Autodesk Fusion 360 part; units mm, degrees
(part 2 of 2)
  constraint coincident L91.end L95
  constraint collinear L91 L92
  constraint collinear L93 L94
  constraint coincident L95.end L99
  constraint collinear L95 L96
  constraint collinear L97 L98
  constraint collinear L99 L100
  constraint coincident L102.start L107
  constraint collinear L101 L102
  constraint coincident L104.start L105
  constraint collinear L103 L104
  constraint collinear L105 L106
  constraint collinear L107 L108
  constraint collinear L109 L110
  constraint collinear L111 L112
  constraint collinear L113 L114
  constraint perpendicular L35 L115
  constraint perpendicular L36 L116
  constraint collinear L341 L342
  constraint coincident L344.start L349
  constraint collinear L343 L344
  constraint coincident L346.start L347
  constraint collinear L345 L346
  constraint collinear L347 L348
  constraint collinear L349 L350
  constraint coincident L351.end L355
  constraint collinear L351 L352
  constraint collinear L353 L354
  constraint coincident L355.end L367
  constraint collinear L355 L356
  constraint coincident L358.start L365
  constraint collinear L357 L358
  constraint coincident L360.start L361
  constraint collinear L359 L360
  constraint coincident A101.end L361
  constraint collinear L361 L362
  constraint collinear L363 L364
  constraint collinear L365 L366
  constraint collinear L367 L368
  constraint coincident L370.start L375
  constraint collinear L369 L370
  constraint coincident L372.start L373
  constraint collinear L371 L372
  constraint collinear L373 L374
  constraint collinear L375 L376
  constraint collinear L377 L378
  constraint coincident L379.end L383
  constraint collinear L379 L380
  constraint coincident L381.end L385
  constraint collinear L381 L382
  constraint collinear L383 L384
  constraint collinear L385 L386
  constraint collinear L387 L388
  constraint coincident L388.start L395
  constraint collinear L389 L390
  constraint coincident L392.start L393
  constraint collinear L391 L392
  constraint collinear L393 L394
  constraint collinear L395 L396
  constraint coincident L398.start L403
  constraint collinear L397 L398
  constraint coincident L400.start L401
  constraint collinear L399 L400
  constraint collinear L401 L402
  constraint collinear L403 L404
  constraint coincident L405.end L409
  constraint collinear L405 L406
  constraint collinear L407 L408
  constraint coincident L409.end L413
  constraint collinear L409 L410
  constraint collinear L411 L412
  constraint collinear L413 L414
  constraint coincident L416.start L423
  constraint collinear L415 L416
  constraint coincident L418.start L421
  constraint collinear L417 L418
  constraint collinear L419 L420
  constraint collinear L421 L422
  constraint collinear L423 L424
  measures "d74" distance of L342.end L352.end
  measures "d82" distance of L341 L355
  measures "d88" diameter of A100
  measures "d89" diameter of A99
  measures "d93" distance of L349 L367
  measures "d95" distance of L341.start L342.end
  measures "d98" distance of A100.centre L367
  measures "d103" distance of L341 L343
  measures "d104" diameter of A97
  measures "d105" diameter of A98
  measures "d106" diameter of A96
  measures "d107" distance of A96.centre L341
  measures "d113" distance of L3.start L3.end
sketch "Schizzo17" plane through (0, 0, 16) normal (0, 0, 1) x (-1, 0, 0) in component "Cubo"
  line L0 (-47.5456, -19.25) -> (-48.649, -19.25)
  arc A0 (-48.649, -18.05) -> (-48.649, -19.25) centre (-49.7456, -18.65) ccw
  line L1 (-48.649, -18.05) -> (-47.5456, -18.05)
  line L2 (-47.5456, -18.05) -> (-47.5456, -12.5)
  line L3 (-47.5456, -12.5) -> (-46.2956, -12.5)
  line L4 (-46.2956, -12.5) -> (-46.2956, -10.9)
  line L5 (-46.2956, -10.9) -> (-48.649, -10.9)
  arc A1 (-48.649, -9.7) -> (-48.649, -10.9) centre (-49.7456, -10.3) ccw
  line L6 (-48.649, -9.7) -> (-46.2956, -9.7)
  line L7 (-46.2956, -9.7) -> (-46.2956, -8.9715)
  arc A2 (-43.6956, -8.9715) -> (-46.2956, -8.9715) centre (-44.9956, -7.8) ccw
  line L8 (-43.6956, -8.9715) -> (-43.6956, -9.7)
  line L9 (-43.6956, -9.7) -> (-41.3421, -9.7)
  arc A3 (-41.3421, -10.9) -> (-41.3421, -9.7) centre (-40.2456, -10.3) ccw
  line L10 (-41.3421, -10.9) -> (-43.6956, -10.9)
  line L11 (-43.6956, -10.9) -> (-43.6956, -12.5)
  line L12 (-43.6956, -12.5) -> (-42.4456, -12.5)
  line L13 (-42.4456, -12.5) -> (-42.4456, -18.05)
  line L14 (-42.4456, -18.05) -> (-41.3421, -18.05)
  arc A4 (-41.3421, -19.25) -> (-41.3421, -18.05) centre (-40.2456, -18.65) ccw
  line L15 (-41.3421, -19.25) -> (-42.4456, -19.25)
  line L16 (-42.4456, -19.25) -> (-42.4456, -24.8)
  line L17 (-42.4456, -24.8) -> (-43.6956, -24.8)
  line L18 (-43.6956, -24.8) -> (-43.6956, -26.4)
  line L19 (-43.6956, -26.4) -> (-41.3421, -26.4)
  arc A5 (-41.3421, -27.6) -> (-41.3421, -26.4) centre (-40.2456, -27) ccw
  line L20 (-41.3421, -27.6) -> (-43.6956, -27.6)
  line L21 (-43.6956, -27.6) -> (-43.6956, -28.3285)
  arc A6 (-46.2956, -28.3285) -> (-43.6956, -28.3285) centre (-44.9956, -29.5) ccw
  line L22 (-46.2956, -28.3285) -> (-46.2956, -27.6)
  line L23 (-46.2956, -27.6) -> (-48.649, -27.6)
  arc A7 (-48.649, -26.4) -> (-48.649, -27.6) centre (-49.7456, -27) ccw
  line L24 (-48.649, -26.4) -> (-46.2956, -26.4)
  line L25 (-46.2956, -26.4) -> (-46.2956, -24.8)
  line L26 (-46.2956, -24.8) -> (-47.5456, -24.8)
  line L27 (-47.5456, -24.8) -> (-47.5456, -19.25)
  arc A8 (-27.7171, -37.25) -> (-27.7171, -36.05) centre (-26.6206, -36.65) ccw
  line L28 (-27.7171, -37.25) -> (-30.0706, -37.25)
  line L29 (-30.0706, -37.25) -> (-30.0706, -38.85)
  line L30 (-30.0706, -38.85) -> (-28.8206, -38.85)
  line L31 (-28.8206, -38.85) -> (-28.8206, -44.4)
  line L32 (-28.8206, -44.4) -> (-27.7171, -44.4)
  arc A9 (-27.7171, -45.6) -> (-27.7171, -44.4) centre (-26.6206, -45) ccw
  line L33 (-27.7171, -45.6) -> (-28.8206, -45.6)
  line L34 (-28.8206, -45.6) -> (-28.8206, -51.15)
  line L35 (-28.8206, -51.15) -> (-30.0706, -51.15)
  line L36 (-30.0706, -51.15) -> (-30.0706, -52.75)
  line L37 (-30.0706, -52.75) -> (-27.7171, -52.75)
  arc A10 (-27.7171, -53.95) -> (-27.7171, -52.75) centre (-26.6206, -53.35) ccw
  line L38 (-27.7171, -53.95) -> (-30.0706, -53.95)
  line L39 (-30.0706, -53.95) -> (-30.0706, -54.6785)
  arc A11 (-32.6706, -54.6785) -> (-30.0706, -54.6785) centre (-31.3706, -55.85) ccw
  line L40 (-32.6706, -54.6785) -> (-32.6706, -53.95)
  line L41 (-32.6706, -53.95) -> (-35.024, -53.95)
  arc A12 (-35.024, -52.75) -> (-35.024, -53.95) centre (-36.1206, -53.35) ccw
  line L42 (-35.024, -52.75) -> (-32.6706, -52.75)
  line L43 (-32.6706, -52.75) -> (-32.6706, -51.15)
  line L44 (-32.6706, -51.15) -> (-33.9206, -51.15)
  line L45 (-33.9206, -51.15) -> (-33.9206, -45.6)
  line L46 (-33.9206, -45.6) -> (-35.024, -45.6)
  arc A13 (-35.024, -44.4) -> (-35.024, -45.6) centre (-36.1206, -45) ccw
  line L47 (-35.024, -44.4) -> (-33.9206, -44.4)
  line L48 (-33.9206, -44.4) -> (-33.9206, -38.85)
  line L49 (-33.9206, -38.85) -> (-32.6706, -38.85)
  line L50 (-32.6706, -38.85) -> (-32.6706, -37.25)
  line L51 (-32.6706, -37.25) -> (-35.024, -37.25)
  arc A14 (-35.024, -36.05) -> (-35.024, -37.25) centre (-36.1206, -36.65) ccw
  line L52 (-35.024, -36.05) -> (-32.6706, -36.05)
  line L53 (-32.6706, -36.05) -> (-32.6706, -35.3215)
  arc A15 (-30.0706, -35.3215) -> (-32.6706, -35.3215) centre (-31.3706, -34.15) ccw
  line L54 (-30.0706, -35.3215) -> (-30.0706, -36.05)
  line L55 (-30.0706, -36.05) -> (-27.7171, -36.05)
  line L56 (-70.9456, -79.1) -> (-68.5921, -79.1)
  arc A16 (-68.5921, -80.3) -> (-68.5921, -79.1) centre (-67.4956, -79.7) ccw
  line L57 (-68.5921, -80.3) -> (-70.9456, -80.3)
  line L58 (-70.9456, -80.3) -> (-70.9456, -81.0285)
  arc A17 (-73.5456, -81.0285) -> (-70.9456, -81.0285) centre (-72.2456, -82.2) ccw
  line L59 (-73.5456, -81.0285) -> (-73.5456, -80.3)
  line L60 (-73.5456, -80.3) -> (-75.899, -80.3)
  arc A18 (-75.899, -79.1) -> (-75.899, -80.3) centre (-76.9956, -79.7) ccw
  line L61 (-75.899, -79.1) -> (-73.5456, -79.1)
  line L62 (-73.5456, -79.1) -> (-73.5456, -77.5)
  line L63 (-73.5456, -77.5) -> (-74.7956, -77.5)
  line L64 (-74.7956, -77.5) -> (-74.7956, -71.95)
  line L65 (-74.7956, -71.95) -> (-75.899, -71.95)
  arc A19 (-75.899, -70.75) -> (-75.899, -71.95) centre (-76.9956, -71.35) ccw
  line L66 (-75.899, -70.75) -> (-74.7956, -70.75)
  line L67 (-74.7956, -70.75) -> (-74.7956, -65.2)
  line L68 (-74.7956, -65.2) -> (-73.5456, -65.2)
  line L69 (-73.5456, -65.2) -> (-73.5456, -63.6)
  line L70 (-73.5456, -63.6) -> (-75.899, -63.6)
  arc A20 (-75.899, -62.4) -> (-75.899, -63.6) centre (-76.9956, -63) ccw
  line L71 (-75.899, -62.4) -> (-73.5456, -62.4)
  line L72 (-73.5456, -62.4) -> (-73.5456, -61.6715)
  arc A21 (-70.9456, -61.6715) -> (-73.5456, -61.6715) centre (-72.2456, -60.5) ccw
  line L73 (-70.9456, -61.6715) -> (-70.9456, -62.4)
  line L74 (-70.9456, -62.4) -> (-68.5921, -62.4)
  arc A22 (-68.5921, -63.6) -> (-68.5921, -62.4) centre (-67.4956, -63) ccw
  line L75 (-68.5921, -63.6) -> (-70.9456, -63.6)
  line L76 (-70.9456, -63.6) -> (-70.9456, -65.2)
  line L77 (-70.9456, -65.2) -> (-69.6956, -65.2)
  line L78 (-69.6956, -65.2) -> (-69.6956, -70.75)
  line L79 (-69.6956, -70.75) -> (-68.5921, -70.75)
  arc A23 (-68.5921, -71.95) -> (-68.5921, -70.75) centre (-67.4956, -71.35) ccw
  line L80 (-68.5921, -71.95) -> (-69.6956, -71.95)
  line L81 (-69.6956, -71.95) -> (-69.6956, -77.5)
  line L82 (-69.6956, -77.5) -> (-70.9456, -77.5)
  line L83 (-70.9456, -77.5) -> (-70.9456, -79.1)
  line L84 (-15.1956, -70.75) -> (-14.0921, -70.75)
  arc A24 (-14.0921, -71.95) -> (-14.0921, -70.75) centre (-12.9956, -71.35) ccw
  line L85 (-14.0921, -71.95) -> (-15.1956, -71.95)
  line L86 (-15.1956, -71.95) -> (-15.1956, -77.5)
  line L87 (-15.1956, -77.5) -> (-16.4456, -77.5)
  line L88 (-16.4456, -77.5) -> (-16.4456, -79.1)
  line L89 (-16.4456, -79.1) -> (-14.0921, -79.1)
  arc A25 (-14.0921, -80.3) -> (-14.0921, -79.1) centre (-12.9956, -79.7) ccw
  line L90 (-14.0921, -80.3) -> (-16.4456, -80.3)
  line L91 (-16.4456, -80.3) -> (-16.4456, -81.0285)
  arc A26 (-19.0456, -81.0285) -> (-16.4456, -81.0285) centre (-17.7456, -82.2) ccw
  line L92 (-19.0456, -81.0285) -> (-19.0456, -80.3)
  line L93 (-19.0456, -80.3) -> (-21.399, -80.3)
  arc A27 (-21.399, -79.1) -> (-21.399, -80.3) centre (-22.4956, -79.7) ccw
  line L94 (-21.399, -79.1) -> (-19.0456, -79.1)
  line L95 (-19.0456, -79.1) -> (-19.0456, -77.5)
  line L96 (-19.0456, -77.5) -> (-20.2956, -77.5)
  line L97 (-20.2956, -77.5) -> (-20.2956, -71.95)
  line L98 (-20.2956, -71.95) -> (-21.399, -71.95)
  arc A28 (-21.399, -70.75) -> (-21.399, -71.95) centre (-22.4956, -71.35) ccw
  line L99 (-21.399, -70.75) -> (-20.2956, -70.75)
  line L100 (-20.2956, -70.75) -> (-20.2956, -65.2)
  line L101 (-20.2956, -65.2) -> (-19.0456, -65.2)
  line L102 (-19.0456, -65.2) -> (-19.0456, -63.6)
  line L103 (-19.0456, -63.6) -> (-21.399, -63.6)
  arc A29 (-21.399, -62.4) -> (-21.399, -63.6) centre (-22.4956, -63) ccw
  line L104 (-21.399, -62.4) -> (-19.0456, -62.4)
  line L105 (-19.0456, -62.4) -> (-19.0456, -61.6715)
  arc A30 (-16.4456, -61.6715) -> (-19.0456, -61.6715) centre (-17.7456, -60.5) ccw
  line L106 (-16.4456, -61.6715) -> (-16.4456, -62.4)
  line L107 (-16.4456, -62.4) -> (-14.0921, -62.4)
  arc A31 (-14.0921, -63.6) -> (-14.0921, -62.4) centre (-12.9956, -63) ccw
  line L108 (-14.0921, -63.6) -> (-16.4456, -63.6)
  line L109 (-16.4456, -63.6) -> (-16.4456, -65.2)
  line L110 (-16.4456, -65.2) -> (-15.1956, -65.2)
  line L111 (-15.1956, -65.2) -> (-15.1956, -70.75)
  line L112 (-57.3206, -62.4) -> (-54.9671, -62.4)
  arc A32 (-54.9671, -63.6) -> (-54.9671, -62.4) centre (-53.8706, -63) ccw
  line L113 (-54.9671, -63.6) -> (-57.3206, -63.6)
  line L114 (-57.3206, -63.6) -> (-57.3206, -65.2)
  line L115 (-57.3206, -65.2) -> (-56.0706, -65.2)
  line L116 (-56.0706, -65.2) -> (-56.0706, -70.75)
  line L117 (-56.0706, -70.75) -> (-54.9671, -70.75)
  arc A33 (-54.9671, -71.95) -> (-54.9671, -70.75) centre (-53.8706, -71.35) ccw
  line L118 (-54.9671, -71.95) -> (-56.0706, -71.95)
  line L119 (-56.0706, -71.95) -> (-56.0706, -77.5)
  line L120 (-56.0706, -77.5) -> (-57.3206, -77.5)
  line L121 (-57.3206, -77.5) -> (-57.3206, -79.1)
  line L122 (-57.3206, -79.1) -> (-54.9671, -79.1)
  arc A34 (-54.9671, -80.3) -> (-54.9671, -79.1) centre (-53.8706, -79.7) ccw
  line L123 (-54.9671, -80.3) -> (-57.3206, -80.3)
  line L124 (-57.3206, -80.3) -> (-57.3206, -81.0285)
  arc A35 (-59.9206, -81.0285) -> (-57.3206, -81.0285) centre (-58.6206, -82.2) ccw
  line L125 (-59.9206, -81.0285) -> (-59.9206, -80.3)
  line L126 (-59.9206, -80.3) -> (-62.274, -80.3)
  arc A36 (-62.274, -79.1) -> (-62.274, -80.3) centre (-63.3706, -79.7) ccw
  line L127 (-62.274, -79.1) -> (-59.9206, -79.1)
  line L128 (-59.9206, -79.1) -> (-59.9206, -77.5)
  line L129 (-59.9206, -77.5) -> (-61.1706, -77.5)
  line L130 (-61.1706, -77.5) -> (-61.1706, -71.95)
  line L131 (-61.1706, -71.95) -> (-62.274, -71.95)
  arc A37 (-62.274, -70.75) -> (-62.274, -71.95) centre (-63.3706, -71.35) ccw
  line L132 (-62.274, -70.75) -> (-61.1706, -70.75)
  line L133 (-61.1706, -70.75) -> (-61.1706, -65.2)
  line L134 (-61.1706, -65.2) -> (-59.9206, -65.2)
  line L135 (-59.9206, -65.2) -> (-59.9206, -63.6)
  line L136 (-59.9206, -63.6) -> (-62.274, -63.6)
  arc A38 (-62.274, -62.4) -> (-62.274, -63.6) centre (-63.3706, -63) ccw
  line L137 (-62.274, -62.4) -> (-59.9206, -62.4)
  line L138 (-59.9206, -62.4) -> (-59.9206, -61.6715)
  arc A39 (-57.3206, -61.6715) -> (-59.9206, -61.6715) centre (-58.6206, -60.5) ccw
  line L139 (-57.3206, -61.6715) -> (-57.3206, -62.4)
  line L140 (-47.5456, -45.6) -> (-48.649, -45.6)
  arc A40 (-48.649, -44.4) -> (-48.649, -45.6) centre (-49.7456, -45) ccw
  line L141 (-48.649, -44.4) -> (-47.5456, -44.4)
  line L142 (-47.5456, -44.4) -> (-47.5456, -38.85)
  line L143 (-47.5456, -38.85) -> (-46.2956, -38.85)
  line L144 (-46.2956, -38.85) -> (-46.2956, -37.25)
  line L145 (-46.2956, -37.25) -> (-48.649, -37.25)
  arc A41 (-48.649, -36.05) -> (-48.649, -37.25) centre (-49.7456, -36.65) ccw
  line L146 (-48.649, -36.05) -> (-46.2956, -36.05)
  line L147 (-46.2956, -36.05) -> (-46.2956, -35.3215)
  arc A42 (-43.6956, -35.3215) -> (-46.2956, -35.3215) centre (-44.9956, -34.15) ccw
  line L148 (-43.6956, -35.3215) -> (-43.6956, -36.05)
  line L149 (-43.6956, -36.05) -> (-41.3421, -36.05)
  arc A43 (-41.3421, -37.25) -> (-41.3421, -36.05) centre (-40.2456, -36.65) ccw
  line L150 (-41.3421, -37.25) -> (-43.6956, -37.25)
  line L151 (-43.6956, -37.25) -> (-43.6956, -38.85)
  line L152 (-43.6956, -38.85) -> (-42.4456, -38.85)
  line L153 (-42.4456, -38.85) -> (-42.4456, -44.4)
  line L154 (-42.4456, -44.4) -> (-41.3421, -44.4)
  arc A44 (-41.3421, -45.6) -> (-41.3421, -44.4) centre (-40.2456, -45) ccw
  line L155 (-41.3421, -45.6) -> (-42.4456, -45.6)
  line L156 (-42.4456, -45.6) -> (-42.4456, -51.15)
  line L157 (-42.4456, -51.15) -> (-43.6956, -51.15)
  line L158 (-43.6956, -51.15) -> (-43.6956, -52.75)
  line L159 (-43.6956, -52.75) -> (-41.3421, -52.75)
  arc A45 (-41.3421, -53.95) -> (-41.3421, -52.75) centre (-40.2456, -53.35) ccw
  line L160 (-41.3421, -53.95) -> (-43.6956, -53.95)
  line L161 (-43.6956, -53.95) -> (-43.6956, -54.6785)
  arc A46 (-46.2956, -54.6785) -> (-43.6956, -54.6785) centre (-44.9956, -55.85) ccw
  line L162 (-46.2956, -54.6785) -> (-46.2956, -53.95)
  line L163 (-46.2956, -53.95) -> (-48.649, -53.95)
  arc A47 (-48.649, -52.75) -> (-48.649, -53.95) centre (-49.7456, -53.35) ccw
  line L164 (-48.649, -52.75) -> (-46.2956, -52.75)
  line L165 (-46.2956, -52.75) -> (-46.2956, -51.15)
  line L166 (-46.2956, -51.15) -> (-47.5456, -51.15)
  line L167 (-47.5456, -51.15) -> (-47.5456, -45.6)
  arc A48 (-27.7171, -10.9) -> (-27.7171, -9.7) centre (-26.6206, -10.3) ccw
  line L168 (-27.7171, -10.9) -> (-30.0706, -10.9)
  line L169 (-30.0706, -10.9) -> (-30.0706, -12.5)
  line L170 (-30.0706, -12.5) -> (-28.8206, -12.5)
  line L171 (-28.8206, -12.5) -> (-28.8206, -18.05)
  line L172 (-28.8206, -18.05) -> (-27.7171, -18.05)
  arc A49 (-27.7171, -19.25) -> (-27.7171, -18.05) centre (-26.6206, -18.65) ccw
  line L173 (-27.7171, -19.25) -> (-28.8206, -19.25)
  line L174 (-28.8206, -19.25) -> (-28.8206, -24.8)
  line L175 (-28.8206, -24.8) -> (-30.0706, -24.8)
  line L176 (-30.0706, -24.8) -> (-30.0706, -26.4)
  line L177 (-30.0706, -26.4) -> (-27.7171, -26.4)
  arc A50 (-27.7171, -27.6) -> (-27.7171, -26.4) centre (-26.6206, -27) ccw
  line L178 (-27.7171, -27.6) -> (-30.0706, -27.6)
  line L179 (-30.0706, -27.6) -> (-30.0706, -28.3285)
  arc A51 (-32.6706, -28.3285) -> (-30.0706, -28.3285) centre (-31.3706, -29.5) ccw
  line L180 (-32.6706, -28.3285) -> (-32.6706, -27.6)
  line L181 (-32.6706, -27.6) -> (-35.024, -27.6)
  arc A52 (-35.024, -26.4) -> (-35.024, -27.6) centre (-36.1206, -27) ccw
  line L182 (-35.024, -26.4) -> (-32.6706, -26.4)
  line L183 (-32.6706, -26.4) -> (-32.6706, -24.8)
  line L184 (-32.6706, -24.8) -> (-33.9206, -24.8)
  line L185 (-33.9206, -24.8) -> (-33.9206, -19.25)
  line L186 (-33.9206, -19.25) -> (-35.024, -19.25)
  arc A53 (-35.024, -18.05) -> (-35.024, -19.25) centre (-36.1206, -18.65) ccw
  line L187 (-35.024, -18.05) -> (-33.9206, -18.05)
  line L188 (-33.9206, -18.05) -> (-33.9206, -12.5)
  line L189 (-33.9206, -12.5) -> (-32.6706, -12.5)
  line L190 (-32.6706, -12.5) -> (-32.6706, -10.9)
  line L191 (-32.6706, -10.9) -> (-35.024, -10.9)
  arc A54 (-35.024, -9.7) -> (-35.024, -10.9) centre (-36.1206, -10.3) ccw
  line L192 (-35.024, -9.7) -> (-32.6706, -9.7)
  line L193 (-32.6706, -9.7) -> (-32.6706, -8.9715)
  arc A55 (-30.0706, -8.9715) -> (-32.6706, -8.9715) centre (-31.3706, -7.8) ccw
  line L194 (-30.0706, -8.9715) -> (-30.0706, -9.7)
  line L195 (-30.0706, -9.7) -> (-27.7171, -9.7)
  line L196 (-59.9206, -27.6) -> (-62.274, -27.6)
  arc A56 (-62.274, -26.4) -> (-62.274, -27.6) centre (-63.3706, -27) ccw
  line L197 (-62.274, -26.4) -> (-59.9206, -26.4)
  line L198 (-59.9206, -26.4) -> (-59.9206, -24.8)
  line L199 (-59.9206, -24.8) -> (-61.1706, -24.8)
  line L200 (-61.1706, -24.8) -> (-61.1706, -19.25)
  line L201 (-61.1706, -19.25) -> (-62.274, -19.25)
  arc A57 (-62.274, -18.05) -> (-62.274, -19.25) centre (-63.3706, -18.65) ccw
  line L202 (-62.274, -18.05) -> (-61.1706, -18.05)
  line L203 (-61.1706, -18.05) -> (-61.1706, -12.5)
  line L204 (-61.1706, -12.5) -> (-59.9206, -12.5)
  line L205 (-59.9206, -12.5) -> (-59.9206, -10.9)
  line L206 (-59.9206, -10.9) -> (-62.274, -10.9)
  arc A58 (-62.274, -9.7) -> (-62.274, -10.9) centre (-63.3706, -10.3) ccw
  line L207 (-62.274, -9.7) -> (-59.9206, -9.7)
  line L208 (-59.9206, -9.7) -> (-59.9206, -8.9715)
  arc A59 (-57.3206, -8.9715) -> (-59.9206, -8.9715) centre (-58.6206, -7.8) ccw
  line L209 (-57.3206, -8.9715) -> (-57.3206, -9.7)
  line L210 (-57.3206, -9.7) -> (-54.9671, -9.7)
  arc A60 (-54.9671, -10.9) -> (-54.9671, -9.7) centre (-53.8706, -10.3) ccw
  line L211 (-54.9671, -10.9) -> (-57.3206, -10.9)
  line L212 (-57.3206, -10.9) -> (-57.3206, -12.5)
  line L213 (-57.3206, -12.5) -> (-56.0706, -12.5)
  line L214 (-56.0706, -12.5) -> (-56.0706, -18.05)
  line L215 (-56.0706, -18.05) -> (-54.9671, -18.05)
  arc A61 (-54.9671, -19.25) -> (-54.9671, -18.05) centre (-53.8706, -18.65) ccw
  line L216 (-54.9671, -19.25) -> (-56.0706, -19.25)
  line L217 (-56.0706, -19.25) -> (-56.0706, -24.8)
  line L218 (-56.0706, -24.8) -> (-57.3206, -24.8)
  line L219 (-57.3206, -24.8) -> (-57.3206, -26.4)
  line L220 (-57.3206, -26.4) -> (-54.9671, -26.4)
  arc A62 (-54.9671, -27.6) -> (-54.9671, -26.4) centre (-53.8706, -27) ccw
  line L221 (-54.9671, -27.6) -> (-57.3206, -27.6)
  line L222 (-57.3206, -27.6) -> (-57.3206, -28.3285)
  arc A63 (-59.9206, -28.3285) -> (-57.3206, -28.3285) centre (-58.6206, -29.5) ccw
  line L223 (-59.9206, -28.3285) -> (-59.9206, -27.6)
  line L224 (-16.4456, -36.05) -> (-14.0921, -36.05)
  arc A64 (-14.0921, -37.25) -> (-14.0921, -36.05) centre (-12.9956, -36.65) ccw
  line L225 (-14.0921, -37.25) -> (-16.4456, -37.25)
  line L226 (-16.4456, -37.25) -> (-16.4456, -38.85)
  line L227 (-16.4456, -38.85) -> (-15.1956, -38.85)
  line L228 (-15.1956, -38.85) -> (-15.1956, -44.4)
  line L229 (-15.1956, -44.4) -> (-14.0921, -44.4)
  arc A65 (-14.0921, -45.6) -> (-14.0921, -44.4) centre (-12.9956, -45) ccw
  line L230 (-14.0921, -45.6) -> (-15.1956, -45.6)
  line L231 (-15.1956, -45.6) -> (-15.1956, -51.15)
  line L232 (-15.1956, -51.15) -> (-16.4456, -51.15)
  line L233 (-16.4456, -51.15) -> (-16.4456, -52.75)
  line L234 (-16.4456, -52.75) -> (-14.0921, -52.75)
  arc A66 (-14.0921, -53.95) -> (-14.0921, -52.75) centre (-12.9956, -53.35) ccw
  line L235 (-14.0921, -53.95) -> (-16.4456, -53.95)
  line L236 (-16.4456, -53.95) -> (-16.4456, -54.6785)
  arc A67 (-19.0456, -54.6785) -> (-16.4456, -54.6785) centre (-17.7456, -55.85) ccw
  line L237 (-19.0456, -54.6785) -> (-19.0456, -53.95)
  line L238 (-19.0456, -53.95) -> (-21.399, -53.95)
  arc A68 (-21.399, -52.75) -> (-21.399, -53.95) centre (-22.4956, -53.35) ccw
  line L239 (-21.399, -52.75) -> (-19.0456, -52.75)
  line L240 (-19.0456, -52.75) -> (-19.0456, -51.15)
  line L241 (-19.0456, -51.15) -> (-20.2956, -51.15)
  line L242 (-20.2956, -51.15) -> (-20.2956, -45.6)
  line L243 (-20.2956, -45.6) -> (-21.399, -45.6)
  arc A69 (-21.399, -44.4) -> (-21.399, -45.6) centre (-22.4956, -45) ccw
  line L244 (-21.399, -44.4) -> (-20.2956, -44.4)
  line L245 (-20.2956, -44.4) -> (-20.2956, -38.85)
  line L246 (-20.2956, -38.85) -> (-19.0456, -38.85)
  line L247 (-19.0456, -38.85) -> (-19.0456, -37.25)
  line L248 (-19.0456, -37.25) -> (-21.399, -37.25)
  arc A70 (-21.399, -36.05) -> (-21.399, -37.25) centre (-22.4956, -36.65) ccw
  line L249 (-21.399, -36.05) -> (-19.0456, -36.05)
  line L250 (-19.0456, -36.05) -> (-19.0456, -35.3215)
  arc A71 (-16.4456, -35.3215) -> (-19.0456, -35.3215) centre (-17.7456, -34.15) ccw
  line L251 (-16.4456, -35.3215) -> (-16.4456, -36.05)
  arc A72 (-68.5921, -37.25) -> (-68.5921, -36.05) centre (-67.4956, -36.65) ccw
  line L252 (-68.5921, -37.25) -> (-70.9456, -37.25)
  line L253 (-70.9456, -37.25) -> (-70.9456, -38.85)
  line L254 (-70.9456, -38.85) -> (-69.6956, -38.85)
  line L255 (-69.6956, -38.85) -> (-69.6956, -44.4)
  line L256 (-69.6956, -44.4) -> (-68.5921, -44.4)
  arc A73 (-68.5921, -45.6) -> (-68.5921, -44.4) centre (-67.4956, -45) ccw
  line L257 (-68.5921, -45.6) -> (-69.6956, -45.6)
  line L258 (-69.6956, -45.6) -> (-69.6956, -51.15)
  line L259 (-69.6956, -51.15) -> (-70.9456, -51.15)
  line L260 (-70.9456, -51.15) -> (-70.9456, -52.75)
  line L261 (-70.9456, -52.75) -> (-68.5921, -52.75)
  arc A74 (-68.5921, -53.95) -> (-68.5921, -52.75) centre (-67.4956, -53.35) ccw
  line L262 (-68.5921, -53.95) -> (-70.9456, -53.95)
  line L263 (-70.9456, -53.95) -> (-70.9456, -54.6785)
  arc A75 (-73.5456, -54.6785) -> (-70.9456, -54.6785) centre (-72.2456, -55.85) ccw
  line L264 (-73.5456, -54.6785) -> (-73.5456, -53.95)
  line L265 (-73.5456, -53.95) -> (-75.899, -53.95)
  arc A76 (-75.899, -52.75) -> (-75.899, -53.95) centre (-76.9956, -53.35) ccw
  line L266 (-75.899, -52.75) -> (-73.5456, -52.75)
  line L267 (-73.5456, -52.75) -> (-73.5456, -51.15)
  line L268 (-73.5456, -51.15) -> (-74.7956, -51.15)
  line L269 (-74.7956, -51.15) -> (-74.7956, -45.6)
  line L270 (-74.7956, -45.6) -> (-75.899, -45.6)
  arc A77 (-75.899, -44.4) -> (-75.899, -45.6) centre (-76.9956, -45) ccw
  line L271 (-75.899, -44.4) -> (-74.7956, -44.4)
  line L272 (-74.7956, -44.4) -> (-74.7956, -38.85)
  line L273 (-74.7956, -38.85) -> (-73.5456, -38.85)
  line L274 (-73.5456, -38.85) -> (-73.5456, -37.25)
  line L275 (-73.5456, -37.25) -> (-75.899, -37.25)
  arc A78 (-75.899, -36.05) -> (-75.899, -37.25) centre (-76.9956, -36.65) ccw
  line L276 (-75.899, -36.05) -> (-73.5456, -36.05)
  line L277 (-73.5456, -36.05) -> (-73.5456, -35.3215)
  arc A79 (-70.9456, -35.3215) -> (-73.5456, -35.3215) centre (-72.2456, -34.15) ccw
  line L278 (-70.9456, -35.3215) -> (-70.9456, -36.05)
  line L279 (-70.9456, -36.05) -> (-68.5921, -36.05)
  line L280 (-32.6706, -80.3) -> (-35.024, -80.3)
  arc A80 (-35.024, -79.1) -> (-35.024, -80.3) centre (-36.1206, -79.7) ccw
  line L281 (-35.024, -79.1) -> (-32.6706, -79.1)
  line L282 (-32.6706, -79.1) -> (-32.6706, -77.5)
  line L283 (-32.6706, -77.5) -> (-33.9206, -77.5)
  line L284 (-33.9206, -77.5) -> (-33.9206, -71.95)
  line L285 (-33.9206, -71.95) -> (-35.024, -71.95)
  arc A81 (-35.024, -70.75) -> (-35.024, -71.95) centre (-36.1206, -71.35) ccw
  line L286 (-35.024, -70.75) -> (-33.9206, -70.75)
  line L287 (-33.9206, -70.75) -> (-33.9206, -65.2)
  line L288 (-33.9206, -65.2) -> (-32.6706, -65.2)
  line L289 (-32.6706, -65.2) -> (-32.6706, -63.6)
  line L290 (-32.6706, -63.6) -> (-35.024, -63.6)
  arc A82 (-35.024, -62.4) -> (-35.024, -63.6) centre (-36.1206, -63) ccw
  line L291 (-35.024, -62.4) -> (-32.6706, -62.4)
  line L292 (-32.6706, -62.4) -> (-32.6706, -61.6715)
  arc A83 (-30.0706, -61.6715) -> (-32.6706, -61.6715) centre (-31.3706, -60.5) ccw
  line L293 (-30.0706, -61.6715) -> (-30.0706, -62.4)
  line L294 (-30.0706, -62.4) -> (-27.7171, -62.4)
  arc A84 (-27.7171, -63.6) -> (-27.7171, -62.4) centre (-26.6206, -63) ccw
  line L295 (-27.7171, -63.6) -> (-30.0706, -63.6)
  line L296 (-30.0706, -63.6) -> (-30.0706, -65.2)
  line L297 (-30.0706, -65.2) -> (-28.8206, -65.2)
  line L298 (-28.8206, -65.2) -> (-28.8206, -70.75)
  line L299 (-28.8206, -70.75) -> (-27.7171, -70.75)
  arc A85 (-27.7171, -71.95) -> (-27.7171, -70.75) centre (-26.6206, -71.35) ccw
  line L300 (-27.7171, -71.95) -> (-28.8206, -71.95)
  line L301 (-28.8206, -71.95) -> (-28.8206, -77.5)
  line L302 (-28.8206, -77.5) -> (-30.0706, -77.5)
  line L303 (-30.0706, -77.5) -> (-30.0706, -79.1)
  line L304 (-30.0706, -79.1) -> (-27.7171, -79.1)
  arc A86 (-27.7171, -80.3) -> (-27.7171, -79.1) centre (-26.6206, -79.7) ccw
  line L305 (-27.7171, -80.3) -> (-30.0706, -80.3)
  line L306 (-30.0706, -80.3) -> (-30.0706, -81.0285)
  arc A87 (-32.6706, -81.0285) -> (-30.0706, -81.0285) centre (-31.3706, -82.2) ccw
  line L307 (-32.6706, -81.0285) -> (-32.6706, -80.3)
  arc A88 (-46.2956, -81.0285) -> (-43.6956, -81.0285) centre (-44.9956, -82.2) ccw
  line L308 (-46.2956, -81.0285) -> (-46.2956, -80.3)
  line L309 (-46.2956, -80.3) -> (-48.649, -80.3)
  arc A89 (-48.649, -79.1) -> (-48.649, -80.3) centre (-49.7456, -79.7) ccw
  line L310 (-48.649, -79.1) -> (-46.2956, -79.1)
  line L311 (-46.2956, -79.1) -> (-46.2956, -77.5)
  line L312 (-46.2956, -77.5) -> (-47.5456, -77.5)
  line L313 (-47.5456, -77.5) -> (-47.5456, -71.95)
  line L314 (-47.5456, -71.95) -> (-48.649, -71.95)
  arc A90 (-48.649, -70.75) -> (-48.649, -71.95) centre (-49.7456, -71.35) ccw
  line L315 (-48.649, -70.75) -> (-47.5456, -70.75)
  line L316 (-47.5456, -70.75) -> (-47.5456, -65.2)
  line L317 (-47.5456, -65.2) -> (-46.2956, -65.2)
  line L318 (-46.2956, -65.2) -> (-46.2956, -63.6)
  line L319 (-46.2956, -63.6) -> (-48.649, -63.6)
  arc A91 (-48.649, -62.4) -> (-48.649, -63.6) centre (-49.7456, -63) ccw
  line L320 (-48.649, -62.4) -> (-46.2956, -62.4)
  line L321 (-46.2956, -62.4) -> (-46.2956, -61.6715)
  arc A92 (-43.6956, -61.6715) -> (-46.2956, -61.6715) centre (-44.9956, -60.5) ccw
  line L322 (-43.6956, -61.6715) -> (-43.6956, -62.4)
  line L323 (-43.6956, -62.4) -> (-41.3421, -62.4)
  arc A93 (-41.3421, -63.6) -> (-41.3421, -62.4) centre (-40.2456, -63) ccw
  line L324 (-41.3421, -63.6) -> (-43.6956, -63.6)
  line L325 (-43.6956, -63.6) -> (-43.6956, -65.2)
  line L326 (-43.6956, -65.2) -> (-42.4456, -65.2)
  line L327 (-42.4456, -65.2) -> (-42.4456, -70.75)
  line L328 (-42.4456, -70.75) -> (-41.3421, -70.75)
  arc A94 (-41.3421, -71.95) -> (-41.3421, -70.75) centre (-40.2456, -71.35) ccw
  line L329 (-41.3421, -71.95) -> (-42.4456, -71.95)
  line L330 (-42.4456, -71.95) -> (-42.4456, -77.5)
  line L331 (-42.4456, -77.5) -> (-43.6956, -77.5)
  line L332 (-43.6956, -77.5) -> (-43.6956, -79.1)
  line L333 (-43.6956, -79.1) -> (-41.3421, -79.1)
  arc A95 (-41.3421, -80.3) -> (-41.3421, -79.1) centre (-40.2456, -79.7) ccw
  line L334 (-41.3421, -80.3) -> (-43.6956, -80.3)
  line L335 (-43.6956, -80.3) -> (-43.6956, -81.0285)
  line L336 (-59.9206, -53.95) -> (-62.274, -53.95)
  arc A96 (-62.274, -52.75) -> (-62.274, -53.95) centre (-63.3706, -53.35) ccw
  line L337 (-62.274, -52.75) -> (-59.9206, -52.75)
  line L338 (-59.9206, -52.75) -> (-59.9206, -51.15)
  line L339 (-59.9206, -51.15) -> (-61.1706, -51.15)
  line L340 (-61.1706, -51.15) -> (-61.1706, -45.6)
  line L341 (-61.1706, -45.6) -> (-62.274, -45.6)
  arc A97 (-62.274, -44.4) -> (-62.274, -45.6) centre (-63.3706, -45) ccw
  line L342 (-62.274, -44.4) -> (-61.1706, -44.4)
  line L343 (-61.1706, -44.4) -> (-61.1706, -38.85)
  line L344 (-61.1706, -38.85) -> (-59.9206, -38.85)
  line L345 (-59.9206, -38.85) -> (-59.9206, -37.25)
  line L346 (-59.9206, -37.25) -> (-62.274, -37.25)
  arc A98 (-62.274, -36.05) -> (-62.274, -37.25) centre (-63.3706, -36.65) ccw
  line L347 (-62.274, -36.05) -> (-59.9206, -36.05)
  line L348 (-59.9206, -36.05) -> (-59.9206, -35.3215)
  arc A99 (-57.3206, -35.3215) -> (-59.9206, -35.3215) centre (-58.6206, -34.15) ccw
  line L349 (-57.3206, -35.3215) -> (-57.3206, -36.05)
  line L350 (-57.3206, -36.05) -> (-54.9671, -36.05)
  arc A100 (-54.9671, -37.25) -> (-54.9671, -36.05) centre (-53.8706, -36.65) ccw
  line L351 (-54.9671, -37.25) -> (-57.3206, -37.25)
  line L352 (-57.3206, -37.25) -> (-57.3206, -38.85)
  line L353 (-57.3206, -38.85) -> (-56.0706, -38.85)
  line L354 (-56.0706, -38.85) -> (-56.0706, -44.4)
  line L355 (-56.0706, -44.4) -> (-54.9671, -44.4)
  arc A101 (-54.9671, -45.6) -> (-54.9671, -44.4) centre (-53.8706, -45) ccw
  line L356 (-54.9671, -45.6) -> (-56.0706, -45.6)
  line L357 (-56.0706, -45.6) -> (-56.0706, -51.15)
  line L358 (-56.0706, -51.15) -> (-57.3206, -51.15)
  line L359 (-57.3206, -51.15) -> (-57.3206, -52.75)
  line L360 (-57.3206, -52.75) -> (-54.9671, -52.75)
  arc A102 (-54.9671, -53.95) -> (-54.9671, -52.75) centre (-53.8706, -53.35) ccw
  line L361 (-54.9671, -53.95) -> (-57.3206, -53.95)
  line L362 (-57.3206, -53.95) -> (-57.3206, -54.6785)
  arc A103 (-59.9206, -54.6785) -> (-57.3206, -54.6785) centre (-58.6206, -55.85) ccw
  line L363 (-59.9206, -54.6785) -> (-59.9206, -53.95)
  arc A104 (-21.399, -9.7) -> (-21.399, -10.9) centre (-22.4956, -10.3) ccw
  line L364 (-21.399, -9.7) -> (-19.0456, -9.7)
  line L365 (-19.0456, -9.7) -> (-19.0456, -8.9715)
  arc A105 (-16.4456, -8.9715) -> (-19.0456, -8.9715) centre (-17.7456, -7.8) ccw
  line L366 (-16.4456, -8.9715) -> (-16.4456, -9.7)
  line L367 (-16.4456, -9.7) -> (-14.0921, -9.7)
  arc A106 (-14.0921, -10.9) -> (-14.0921, -9.7) centre (-12.9956, -10.3) ccw
  line L368 (-14.0921, -10.9) -> (-16.4456, -10.9)
  line L369 (-16.4456, -10.9) -> (-16.4456, -12.5)
  line L370 (-16.4456, -12.5) -> (-15.1956, -12.5)
  line L371 (-15.1956, -12.5) -> (-15.1956, -18.05)
  line L372 (-15.1956, -18.05) -> (-14.0921, -18.05)
  arc A107 (-14.0921, -19.25) -> (-14.0921, -18.05) centre (-12.9956, -18.65) ccw
  line L373 (-14.0921, -19.25) -> (-15.1956, -19.25)
  line L374 (-15.1956, -19.25) -> (-15.1956, -24.8)
  line L375 (-15.1956, -24.8) -> (-16.4456, -24.8)
  line L376 (-16.4456, -24.8) -> (-16.4456, -26.4)
  line L377 (-16.4456, -26.4) -> (-14.0921, -26.4)
  arc A108 (-14.0921, -27.6) -> (-14.0921, -26.4) centre (-12.9956, -27) ccw
  line L378 (-14.0921, -27.6) -> (-16.4456, -27.6)
  line L379 (-16.4456, -27.6) -> (-16.4456, -28.3285)
  arc A109 (-19.0456, -28.3285) -> (-16.4456, -28.3285) centre (-17.7456, -29.5) ccw
  line L380 (-19.0456, -28.3285) -> (-19.0456, -27.6)
  line L381 (-19.0456, -27.6) -> (-21.399, -27.6)
  arc A110 (-21.399, -26.4) -> (-21.399, -27.6) centre (-22.4956, -27) ccw
  line L382 (-21.399, -26.4) -> (-19.0456, -26.4)
  line L383 (-19.0456, -26.4) -> (-19.0456, -24.8)
  line L384 (-19.0456, -24.8) -> (-20.2956, -24.8)
  line L385 (-20.2956, -24.8) -> (-20.2956, -19.25)
  line L386 (-20.2956, -19.25) -> (-21.399, -19.25)
  arc A111 (-21.399, -18.05) -> (-21.399, -19.25) centre (-22.4956, -18.65) ccw
  line L387 (-21.399, -18.05) -> (-20.2956, -18.05)
  line L388 (-20.2956, -18.05) -> (-20.2956, -12.5)
  line L389 (-20.2956, -12.5) -> (-19.0456, -12.5)
  line L390 (-19.0456, -12.5) -> (-19.0456, -10.9)
  line L391 (-19.0456, -10.9) -> (-21.399, -10.9)
  arc A112 (-68.5921, -10.9) -> (-68.5921, -9.7) centre (-67.4956, -10.3) ccw
  line L392 (-68.5921, -10.9) -> (-70.9456, -10.9)
  line L393 (-70.9456, -10.9) -> (-70.9456, -12.5)
  line L394 (-70.9456, -12.5) -> (-69.6956, -12.5)
  line L395 (-69.6956, -12.5) -> (-69.6956, -18.05)
  line L396 (-69.6956, -18.05) -> (-68.5921, -18.05)
  arc A113 (-68.5921, -19.25) -> (-68.5921, -18.05) centre (-67.4956, -18.65) ccw
  line L397 (-68.5921, -19.25) -> (-69.6956, -19.25)
  line L398 (-69.6956, -19.25) -> (-69.6956, -24.8)
  line L399 (-69.6956, -24.8) -> (-70.9456, -24.8)
  line L400 (-70.9456, -24.8) -> (-70.9456, -26.4)
  line L401 (-70.9456, -26.4) -> (-68.5921, -26.4)
  arc A114 (-68.5921, -27.6) -> (-68.5921, -26.4) centre (-67.4956, -27) ccw
  line L402 (-68.5921, -27.6) -> (-70.9456, -27.6)
  line L403 (-70.9456, -27.6) -> (-70.9456, -28.3285)
  arc A115 (-73.5456, -28.3285) -> (-70.9456, -28.3285) centre (-72.2456, -29.5) ccw
  line L404 (-73.5456, -28.3285) -> (-73.5456, -27.6)
  line L405 (-73.5456, -27.6) -> (-75.899, -27.6)
  arc A116 (-75.899, -26.4) -> (-75.899, -27.6) centre (-76.9956, -27) ccw
  line L406 (-75.899, -26.4) -> (-73.5456, -26.4)
  line L407 (-73.5456, -26.4) -> (-73.5456, -24.8)
  line L408 (-73.5456, -24.8) -> (-74.7956, -24.8)
  line L409 (-74.7956, -24.8) -> (-74.7956, -19.25)
  line L410 (-74.7956, -19.25) -> (-75.899, -19.25)
  arc A117 (-75.899, -18.05) -> (-75.899, -19.25) centre (-76.9956, -18.65) ccw
  line L411 (-75.899, -18.05) -> (-74.7956, -18.05)
  line L412 (-74.7956, -18.05) -> (-74.7956, -12.5)
  line L413 (-74.7956, -12.5) -> (-73.5456, -12.5)
  line L414 (-73.5456, -12.5) -> (-73.5456, -10.9)
  line L415 (-73.5456, -10.9) -> (-75.899, -10.9)
  arc A118 (-75.899, -9.7) -> (-75.899, -10.9) centre (-76.9956, -10.3) ccw
  line L416 (-75.899, -9.7) -> (-73.5456, -9.7)
  line L417 (-73.5456, -9.7) -> (-73.5456, -8.9715)
  arc A119 (-70.9456, -8.9715) -> (-73.5456, -8.9715) centre (-72.2456, -7.8) ccw
  line L418 (-70.9456, -8.9715) -> (-70.9456, -9.7)
  line L419 (-70.9456, -9.7) -> (-68.5921, -9.7)
  line L420 (-4, -86) -> (-4, -4)
  line L421 (-4, -4) -> (-86, -4)
  line L422 (-86, -4) -> (-86, -86)
  line L423 (-86, -86) -> (-4, -86)
  line L424 (0, -90) -> (-45, -90)
  line L425 (-45, -90) -> (-45, -95)
  line L426 (0, -90) -> (0, -45)
  line L427 (0, -45) -> (5, -45)
  circle A120 centre (-8, -82) radius 2.75
  circle A121 centre (-82, -82) radius 2.75
  circle A122 centre (-8, -8) radius 2.75
  circle A123 centre (-82, -8) radius 2.75
  dimension "d137" = 45
  dimension "d138" = 45
  dimension "d139" = 5.5
  constraint horizontal L424
  constraint perpendicular L424 L425
  constraint perpendicular L424 L426
  constraint perpendicular L426 L427
  constraint symmetric L425 A120 A121
  constraint symmetric L427 A120 A122
  constraint symmetric L427 A121 A123
  measures "d137" distance of L424.start L424.end
  measures "d138" distance of L424.start L426.end
  measures "d139" diameter of A120
sketch "Schizzo18" plane through (0, 0, 101) normal (0, 0, -1) x (1, 0, 0) in component "Cubo"
  line L0 (-33.5, -3.5) -> (-33.5, -86.5)
  line L1 (-33.5, -86.5) -> (-116.5, -86.5)
  line L2 (-116.5, -86.5) -> (-116.5, -3.5)
  line L3 (-116.5, -3.5) -> (-33.5, -3.5)
  arc A0 (-33, -90) -> (-30, -87) centre (-33, -87) ccw
  line L4 (-30, -87) -> (-30, -3)
  arc A1 (-30, -3) -> (-33, 0) centre (-33, -3) ccw
  line L5 (-33, 0) -> (-117, 0)
  arc A2 (-117, 0) -> (-120, -3) centre (-117, -3) ccw
  line L6 (-120, -3) -> (-120, -87)
  arc A3 (-120, -87) -> (-117, -90) centre (-117, -87) ccw
  line L7 (-117, -90) -> (-33, -90)
  line L8 (-116.5, -3.5) -> (-108, -3.5)
  line L9 (-108, -3.5) -> (-108, -12)
  line L10 (-108, -12) -> (-116.5, -12)
  line L11 (-116.5, -12) -> (-116.5, -3.5)
  circle A4 centre (-112, -8) radius 2.75
  line L12 (-75, 0) -> (-75, 6)
  line L13 (-120, -45) -> (-130, -45)
  line L14 (-33.5, -3.5) -> (-42, -3.5)
  line L15 (-42, -3.5) -> (-42, -12)
  line L16 (-42, -12) -> (-33.5, -12)
  line L17 (-33.5, -12) -> (-33.5, -3.5)
  line L18 (-33.5, -86.5) -> (-42, -86.5)
  line L19 (-42, -86.5) -> (-42, -78)
  line L20 (-42, -78) -> (-33.5, -78)
  line L21 (-33.5, -78) -> (-33.5, -86.5)
  line L22 (-116.5, -86.5) -> (-108, -86.5)
  line L23 (-108, -86.5) -> (-108, -78)
  line L24 (-108, -78) -> (-116.5, -78)
  line L25 (-116.5, -78) -> (-116.5, -86.5)
  dimension "d146" = 5.5
  dimension "d147" = 8
  dimension "d148" = 8
  dimension "d150" = 8.5
  dimension "d151" = 8.5
  dimension "d152" = 8.5
  dimension "d153" = 8.5
  dimension "d154" = 8.5
  dimension "d155" = 8.5
  dimension "d156" = 8.5
  constraint horizontal L8
  constraint vertical L9
  constraint horizontal L10
  constraint vertical L11
  constraint coincident L2.end L3.start
  constraint midpoint L5 L12.start
  constraint perpendicular L5 L12
  constraint midpoint L6 L13.start
  constraint perpendicular L6 L13
  constraint horizontal L14
  constraint vertical L15
  constraint horizontal L16
  constraint vertical L17
  constraint coincident L0.start L3.end
  constraint horizontal L18
  constraint vertical L19
  constraint horizontal L20
  constraint vertical L21
  constraint coincident L0.end L1.start
  constraint horizontal L22
  constraint vertical L23
  constraint horizontal L24
  constraint vertical L25
  constraint coincident L1.end L2.start
  measures "d146" diameter of A4
  measures "d147" distance of L5 A4.centre
  measures "d148" distance of L6 A4.centre
  measures "d150" distance of L8.end L9.end
  measures "d151" distance of L0.start L14.end
  measures "d152" distance of L0.start L16.end
  measures "d153" distance of L0.end L18.end
  measures "d154" distance of L0.end L20.end
  measures "d155" distance of L1.end L22.end
  measures "d156" distance of L1.end L24.end
sketch "Schizzo19" plane through (0, 0, 101) normal (0, 0, -1) x (1, 0, 0) in component "Cubo"
  line L0 (-33.5, -78) -> (-42, -78)
  line L1 (-42, -78) -> (-42, -86.5)
  line L2 (-108, -86.5) -> (-108, -78)
  line L3 (-108, -78) -> (-116.5, -78)
  line L4 (-116.5, -12) -> (-108, -12)
  line L5 (-108, -12) -> (-108, -3.5)
  line L6 (-42, -3.5) -> (-42, -12)
  line L7 (-42, -12) -> (-33.5, -12)
  line L8 (-108, -12) -> (-116.5, -12)
  line L9 (-116.5, -12) -> (-116.5, -3.5)
  line L10 (-116.5, -3.5) -> (-108, -3.5)
  line L11 (-108, -3.5) -> (-108, -12)
  line L12 (-42, -12) -> (-33.5, -12)
  line L13 (-33.5, -12) -> (-33.5, -3.5)
  line L14 (-33.5, -3.5) -> (-42, -3.5)
  line L15 (-42, -3.5) -> (-42, -12)
  line L16 (-42, -78) -> (-33.5, -78)
  line L17 (-33.5, -78) -> (-33.5, -86.5)
  line L18 (-33.5, -86.5) -> (-42, -86.5)
  line L19 (-42, -86.5) -> (-42, -78)
  line L20 (-108, -78) -> (-116.5, -78)
  line L21 (-116.5, -78) -> (-116.5, -86.5)
  line L22 (-116.5, -86.5) -> (-108, -86.5)
  line L23 (-108, -86.5) -> (-108, -78)
  line L24 (-116.5, -78) -> (-116.5, -86.5)
  line L25 (-116.5, -86.5) -> (-108, -86.5)
  line L26 (-33.5, -12) -> (-33.5, -3.5)
  line L27 (-33.5, -3.5) -> (-42, -3.5)
  line L28 (-42, -86.5) -> (-33.5, -86.5)
  line L29 (-33.5, -86.5) -> (-33.5, -78)
  line L30 (-108, -3.5) -> (-116.5, -3.5)
  line L31 (-116.5, -3.5) -> (-116.5, -12)
  dimension "d159" = 8.5
  dimension "d160" = 8.5
  dimension "d161" = 8.5
  dimension "d162" = 8.5
  dimension "d163" = 8.5
  dimension "d164" = 8.5
  dimension "d165" = 8.5
  dimension "d166" = 8.5
  constraint horizontal L8
  constraint vertical L9
  constraint horizontal L10
  constraint vertical L11
  constraint coincident L4.end L5.start
  constraint horizontal L12
  constraint vertical L13
  constraint horizontal L14
  constraint vertical L15
  constraint coincident L6.end L7.start
  constraint horizontal L16
  constraint vertical L17
  constraint horizontal L18
  constraint vertical L19
  constraint coincident L0.end L1.start
  constraint horizontal L20
  constraint vertical L21
  constraint horizontal L22
  constraint vertical L23
  constraint coincident L2.end L3.start
  measures "d159" distance of L4.end L4.start
  measures "d160" distance of L4.end L5.end
  measures "d161" distance of L6.end L7.end
  measures "d162" distance of L6.end L6.start
  measures "d163" distance of L0.end L0.start
  measures "d164" distance of L0.end L1.end
  measures "d165" distance of L2.end L3.end
  measures "d166" distance of L2.end L2.start
sketch "Schizzo20" plane through (0, 0, 106) normal (0, 0, -1) x (1, 0, 0) in component "Cubo"
  circle A0 centre (-112, -8) radius 2.75
  line L0 (-33, 0) -> (-117, 0)
  line L1 (-120, -3) -> (-120, -87)
  line L2 (-75, 0) -> (-75, 5)
  line L3 (-120, -45) -> (-127, -45)
  circle A1 centre (-38, -8) radius 2.75
  circle A2 centre (-112, -82) radius 2.75
  circle A3 centre (-38, -82) radius 2.75
  line L4 (-42, -86.5) -> (-33.5, -86.5)
  line L5 (-33.5, -86.5) -> (-33.5, -78)
  line L6 (-33.5, -78) -> (-42, -78)
  line L7 (-42, -78) -> (-42, -86.5)
  dimension "d169" = 5.5
  dimension "d170" = 8
  dimension "d171" = 8
  constraint midpoint L0 L2.start
  constraint perpendicular L0 L2
  constraint midpoint L1 L3.start
  constraint perpendicular L1 L3
  constraint symmetric A0 L2 A1
  constraint symmetric A0 L3 A2
  constraint symmetric L3 A1 A3
  measures "d169" diameter of A0
  measures "d170" distance of A0.centre L0
  measures "d171" distance of A0.centre L1
sketch "Schizzo1 (2)" plane through (0, 0, 0) normal (0, 0, 1) x (1, 0, 0) in component "Question"
  circle A0 centre (202, 82) radius 2.3
  line L0 (176.2, 64.5828) -> (176.2, 53.4172)
  line L1 (176.2, 53.4172) -> (175.0828, 52.3)
  line L2 (175.0828, 52.3) -> (164.0828, 52.3)
  line L3 (164.0828, 52.3) -> (156.2, 44.4172)
  line L4 (156.2, 44.4172) -> (156.2, 30.0828)
  line L5 (156.2, 30.0828) -> (157.0828, 29.2)
  line L6 (157.0828, 29.2) -> (172.9172, 29.2)
  line L7 (172.9172, 29.2) -> (173.8, 30.0828)
  line L8 (173.8, 30.0828) -> (173.8, 39.5828)
  line L9 (173.8, 39.5828) -> (174.9172, 40.7)
  line L10 (174.9172, 40.7) -> (185.9172, 40.7)
  line L11 (185.9172, 40.7) -> (193.8, 48.5828)
  line L12 (193.8, 48.5828) -> (193.8, 69.4172)
  line L13 (193.8, 69.4172) -> (185.9172, 77.3)
  line L14 (185.9172, 77.3) -> (144.0828, 77.3)
  line L15 (144.0828, 77.3) -> (136.2, 69.4172)
  line L16 (136.2, 69.4172) -> (136.2, 53.5828)
  line L17 (136.2, 53.5828) -> (137.0828, 52.7)
  line L18 (137.0828, 52.7) -> (152.9172, 52.7)
  line L19 (152.9172, 52.7) -> (153.8, 53.5828)
  line L20 (153.8, 53.5828) -> (153.8, 64.5828)
  line L21 (153.8, 64.5828) -> (154.9172, 65.7)
  line L22 (154.9172, 65.7) -> (175.0828, 65.7)
  line L23 (175.0828, 65.7) -> (176.2, 64.5828)
  line L24 (172.9172, 13.2) -> (157.0828, 13.2)
  line L25 (157.0828, 13.2) -> (156.2, 14.0828)
  line L26 (156.2, 14.0828) -> (156.2, 23.9172)
  line L27 (156.2, 23.9172) -> (157.0828, 24.8)
  line L28 (157.0828, 24.8) -> (172.9172, 24.8)
  line L29 (172.9172, 24.8) -> (173.8, 23.9172)
  line L30 (173.8, 23.9172) -> (173.8, 14.0828)
  line L31 (173.8, 14.0828) -> (172.9172, 13.2)
extrude "Estrusione1" add sketch "Schizzo1 (2)" along normal blind 2 makes body 1 at (187.9333, 60.8609, 0) makes body 2 at (162.3609, 17.0667, 0) makes body 3 at (200.0374, 80.8007, 1.3333) in component "Question"
copy_body "Corpo->Comp1" bodies 1 removing the originals makes body 4 in component "Domanda"
copy_body "Corpo->Comp2" bodies 3 removing the originals makes body 5 in component "Dot"
copy_body "Corpo->Comp3" bodies 2 removing the originals makes body 6 in component "Punto"
component "Cubo" placed x (1, 0, 0) y (0, 1, 0) z (0, 0, 1) at (0, 0, 0)
component "Dot" placed x (1, 0, 0) y (0, 1, 0) z (0, 0, 1) at (30, 0, 0)
component "Dot" placed x (1, 0, 0) y (0, 1, 0) z (0, 0, 1) at (0, -70, 0)
component "Dot" placed x (1, 0, 0) y (0, 1, 0) z (0, 0, 1) at (30, -70, 0)
component "Punto" placed x (1, 0, 0) y (0, 1, 0) z (0, 0, 1) at (0, -20, 0)
component "Dot" placed x (1, 0, 0) y (0, 1, 0) z (0, 0, 1) at (0, 0, 0)
component "Domanda" placed x (1, 0, 0) y (0, 1, 0) z (0, 0, 1) at (0, 60, 0)
component "Question" placed x (1, 0, 0) y (0, 1, 0) z (0, 0, 1) at (0, 0, 0) in component "Cubo"
